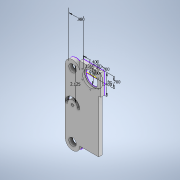
# Autodesk Inventor part: new conveyor bar
Saved by Autodesk Inventor 2021 (Build 250183000, 183)
## iProperties
Created: 2021-01-23
Part Number: new conveyor bar
Material: Generic
Document SubType Name: Modeling
Designer: User
Density: 1 g/cm^3
Appearance: Default
Author: User
Autodesk Inventor part; units mm, degrees
ref_plane "YZ Plane" through (0, 0, 0) normal (1, 0, 0) x (0, 1, 0)
ref_plane "XZ Plane" through (0, 0, 0) normal (0, 1, 0) x (-1, 0, 0)
ref_plane "XY Plane" through (0, 0, 0) normal (0, 0, 1) x (1, 0, 0)
sketch "Sketch1" plane through (0, 0, 0) normal (0, 0, 1) x (1, 0, 0)
  line L0 (0, -93.8479) -> (0, 14.1021) construction
  line L1 (-12.446, -93.8479) -> (-12.446, 14.1021)
  line L2 (12.446, 14.1021) -> (12.446, -93.8479)
  arc A0 (-12.446, -93.8479) -> (12.446, -93.8479) centre (0, -93.8479) ccw
  arc A1 (12.446, 14.1021) -> (-12.446, 14.1021) centre (0, 14.1021) ccw
  point P0 (0, 0)
  point P1 (0, -39.8729)
  dimension "d0" = 53.975
  dimension "d1" = 24.892
  constraints: 8 end point, 4 point on circle, 4 tangent, 2 centre point, 1 midpoint, 1 parallel, 1 vertical
  measures "d0" distance of point (0, -39.873) L0.end
  measures "d1" distance between parallel lines of L2 L1
extrude "Extrusion1" add sketch "Sketch1" along normal blind 6.096
sketch "Sketch2" plane through (0, 0, 6.096) normal (0, 0, 1) x (1, 0, 0)
  line L0 (-12.446, 14.1021) -> (-12.446, -93.8479) projected
  arc A0 (-12.446, -93.8479) -> (12.446, -93.8479) centre (0, -93.8479) ccw projected
  line L1 (12.446, -93.8479) -> (12.446, 14.1021) projected
  arc A1 (12.446, 14.1021) -> (-12.446, 14.1021) centre (0, 14.1021) ccw projected
  point P0 (0, 0)
  point P1 (0, -39.8729)
hole "Hole1" at (0, 14.1021, 6.096) at (0, -93.8479, 6.096) direction (0, 0, -1) diameter 12.7 depth 5.7785 tip angle 118
hole "Hole2" at (0, -39.8729, 0) direction (0, 0, 1) diameter 5.08 depth 5.7785 tip angle 118
sketch "Sketch3" plane through (0, 0, 0) normal (0, 0, -1) x (-1, 0, 0)
  circle A0 centre (0, -39.8729) radius 2.0116 projected
  arc A1 (10, -39.8729) -> (-10, -39.8729) centre (0, -39.8729) ccw construction
  arc A2 (12.032, -39.8729) -> (-12.032, -39.8729) centre (0, -39.8729) ccw
  arc A3 (7.968, -39.8729) -> (-7.968, -39.8729) centre (0, -39.8729) ccw
  arc A4 (7.968, -39.8729) -> (12.032, -39.8729) centre (10, -39.8729) ccw
  arc A5 (-12.032, -39.8729) -> (-7.968, -39.8729) centre (-10, -39.8729) ccw
  point P0 (0, 0)
  dimension "d18" = 2.032
  dimension "d19" = 10
  constraints: 10 point on circle, 5 centre point, 4 tangent, 1 coincident
  measures "d18" radius of A5
  measures "d19" distance of A1.centre A1.end
extrude "Extrusion2" cut sketch "Sketch3" against normal through all contours A4 A3 A5 A2
sketch "Sketch4" plane through (12.446, -93.8479, 0) normal (1, 0, 0) x (0, 0, -1)
  line L0 (0, 0) -> (0, 107.95) projected
  line L1 (0, 107.95) -> (-6.096, 107.95) projected
  line L2 (-6.096, 0) -> (-6.096, 107.95) projected
  line L3 (0, 0) -> (-6.096, 0) projected
  point P0 (0, 93.8479)
extrude "Extrusion3" add sketch "Sketch4" along normal blind 31.75
sketch "Sketch5" plane through (0, 0, 0) normal (0, 0, -1) x (-1, 0, 0)
  line L0 (-12.0232, -4.6927) -> (-47.5832, -4.6927)
  line L1 (-47.5832, -4.6927) -> (-47.5832, 30.8673)
  line L2 (-47.5832, 30.8673) -> (-12.0232, 30.8673)
  line L3 (-12.0232, 30.8673) -> (-12.0232, -4.6927)
  circle A0 centre (-29.8032, 13.0873) radius 12.7
  line L4 (1.5141, 13.0873) -> (-49.7014, 13.0873)
  line L5 (-12.446, 14.1021) -> (-44.196, 14.1021) projected
  point P0 (0, 0)
  point P1 (-29.8032, 28.6575)
  point P2 (-43.2874, 20.8724)
  point P3 (-43.2874, 5.3022)
  point P4 (-29.8032, -2.4829)
  point P5 (-16.3191, 5.3022)
  point P6 (-16.3191, 20.8724)
  point P7 (-47.5832, 13.0873)
  point P8 (-42.5032, 13.0873)
  point P9 (-17.1032, 13.0873)
  point P10 (-12.0232, 13.0873)
  dimension "d24" = 35.56
  dimension "d25" = 35.56
  dimension "d26" = 25.4
  dimension "d27" = 17.78
  dimension "d28" = 17.78
  dimension "d29" = 15.5702
  dimension "d32" = 360
  constraints: 8 end point, 2 parallel, 1 centre point, 1 horizontal, 1 perpendicular, 1 point on line, 1 vertical, 10 other
  measures "d24" distance of L1.end L2.end
  measures "d25" distance of L0.end L1.end
  measures "d26" diameter of A0
  measures "d27" distance from line of L2 A0.centre
  measures "d28" distance from line of L1 A0.centre
  measures "d29" distance of A0.centre point (-29.803, 28.657)
extrude "Extrusion4" add sketch "Sketch5" against normal up to surface (6.096 mm away) contours L0 L1 L4 A0 L3 | L4 A0 L1 L2 L3
extrude "Extrusion5" cut sketch "Sketch5" against normal through all contours L4 A0 L5 | A0 L4 | L5 A0
hole "Hole3" at (16.3191, 20.8724, 0) at (16.3191, 5.3022, 0) at (29.8032, -2.4829, 0) at (43.2874, 5.3022, 0) at (43.2874, 20.8724, 0) at (29.8032, 28.6575, 0) direction (0, 0, 1) diameter 2.3368 depth 5.7785 tip angle 118
equation "\"d27\" = 0.5 * d25"
equation "\"d28\" = 0.5 * d24"
body "Solid1"
